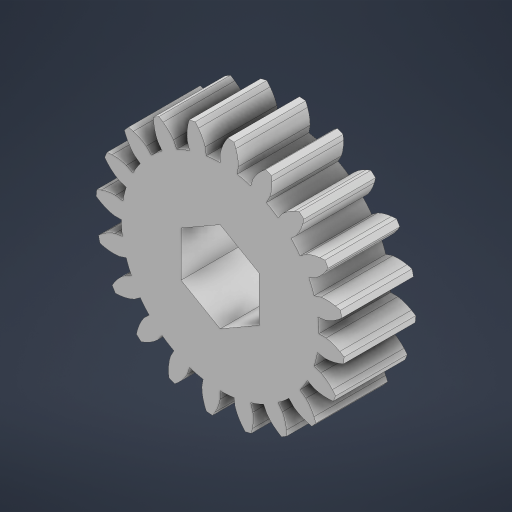
# Autodesk Inventor part: SpurGearTemplate
Saved by Autodesk Inventor 2024 (Build 280153000, 153)
## iProperties
Created: 2023-09-27
Part Number: SpurGearTemplate
Material: Generic
Document SubType Name: Modeling
Designer: avsar
Density: 1 g/cm^3
Appearance: Default
Author: avsar
Autodesk Inventor part; units mm, degrees
ref_plane "YZ Plane" through (0, 0, 0) normal (1, 0, 0) x (0, 1, 0)
ref_plane "XZ Plane" through (0, 0, 0) normal (0, 1, 0) x (-1, 0, 0)
ref_plane "XY Plane" through (0, 0, 0) normal (0, 0, 1) x (1, 0, 0)
sketch "Sketch1" plane through (0, 0, 0) normal (0, 0, 1) x (1, 0, 0)
  circle A0 centre (0, 0) radius 10 construction
  arc A1 (1.2256, 10.9315) -> (1.2111, 10.9331) centre (0, 0) ccw
  arc A2 (8.75, 0) -> (1.5067, 8.6193) centre (0, 0) ccw construction
  circle A3 centre (0, 0) radius 9 construction
  circle A4 centre (0, 0) radius 9.3969 construction
  line L0 (0, 0) -> (0, 9.3969) construction
  line L1 (0, 0) -> (4.6985, 8.138)
  line L2 (0, 0) -> (8.138, 4.6985)
  line L3 (0, 0) -> (9.3969, 0)
  line L4 (9.3969, 0) -> (9.3969, 14.7607) construction
  line L5 (8.138, 4.6985) -> (3.2178, 13.2205) construction
  line L6 (4.6985, 8.138) -> (0.4374, 10.5981) construction
  arc A5 (0.4374, 10.5981) -> (0, 9.3969) centre (3.6283, 8.7558) ccw
  arc A6 (3.2178, 13.2205) -> (0.9898, 11.41) centre (6.2054, 7.268) ccw construction
  arc A7 (9.3969, 14.7607) -> (3.2178, 13.2205) centre (9.7364, 0.2327) ccw construction
  line L7 (0, 0) -> (3.0902, 9.5106)
  line L8 (0, 0) -> (1.5643, 9.8769) construction
  arc A8 (1.5643, 9.8769) -> (0.1598, 9.9987) centre (0, 0) ccw construction
  line L9 (0.8642, 9.9626) -> (0, 0) construction
  arc A9 (3.0902, 9.5106) -> (0.1598, 9.9987) centre (0, 0) ccw construction
  arc A10 (1.6181, 9.2566) -> (1.394, 10.5151) centre (-2.0664, 9.2498) ccw
  arc A11 (1.394, 10.5151) -> (1.2256, 10.9315) centre (-4.8612, 8.2279) ccw
  arc A12 (-0.8932, 13.5771) -> (-6.7149, 16.1583) centre (-9.5509, 1.9057) ccw construction
  arc A13 (5.2789, 9.6506) -> (1.2256, 10.9315) centre (0, 0) ccw construction
  arc A14 (0.675, 10.9793) -> (5.2789, 9.6506) centre (0, 0) ccw construction
  arc A15 (0.9898, 11.41) -> (0.675, 10.9793) centre (6.2054, 7.268) ccw construction
  arc A16 (0.6896, 10.9784) -> (0.675, 10.9793) centre (0, 0) ccw
  arc A17 (1.2111, 10.9331) -> (0.6896, 10.9784) centre (0, 0) ccw
  arc A18 (1.2256, 10.9315) -> (-0.8932, 13.5771) centre (-4.8612, 8.2279) ccw construction
  arc A19 (0.675, 10.9793) -> (0.4374, 10.5981) centre (6.2054, 7.268) ccw
  line L10 (1.6181, 9.2566) -> (0, 0) construction
  arc A20 (0, 8.75) -> (8.75, 0) centre (0, 0) ccw construction
  arc A21 (1.5067, 8.6193) -> (0.7562, 8.7173) centre (0, 0) ccw
  arc A22 (0.7562, 8.7173) -> (0, 8.75) centre (0, 0) ccw
  line L11 (0, 9.3969) -> (0, 8.75)
  line L12 (1.5067, 8.6193) -> (1.6181, 9.2566)
  dimension "BaseCircle" = 18.7938
  dimension "PitchCircle" = 20
  dimension "AddendumCircle" = 22
  dimension "RootCircle" = 17.5
  dimension "ClearanceCircle" = 18
  dimension "InvoluteControl" = 90
  dimension "BaseCircleQuarterCircumference" = 14.7607
  dimension "d10" = 9.8404
  dimension "d11" = 4.9202
  dimension "CircularPitch" = 18
  constraints: 50 point on circle, 26 end point, 22 centre point, 7 symmetric about line, 5 coincident, 5 point on line, 2 collinear, 2 concentric, 2 tangent, 2 vertical, 1 line through centre, 1 vertical alignment, 18 other
  measures "PitchCircle" diameter of A0
  measures "AddendumCircle" diameter of A1
  measures "RootCircle" diameter of A2
  measures "ClearanceCircle" diameter of A3
  measures "BaseCircleQuarterCircumference" distance of L3.end L4.end
  measures "d10" distance of L2.end L5.end
  measures "d11" distance of L1.end L6.end
  measures "CircularPitch" angle of L7 L0
extrude "Extrusion1" add sketch "Sketch1" along normal mid plane 6.35
pattern_circular "Circular Pattern1" count 20 over 360 about axis through (0, 0, -10) along (0, 0, 1) of "Extrusion1"
sketch "Sketch2" plane through (0, 0, 0) normal (0, 0, 1) x (1, 0, 0)
  arc A0 (0, 8.75) -> (8.75, 0) centre (0, 0) ccw construction
  circle A1 centre (0, 0) radius 8.75
  arc A2 (8.75, 0) -> (1.5067, 8.6193) centre (0, 0) ccw construction
  constraints: 1 centre point, 1 coincident, 1 concentric
extrude "Extrusion2" add sketch "Sketch2" along normal mid plane 6.35
sketch "Sketch3" plane through (0, 0, 3.175) normal (0, 0, 1) x (1, 0, 0)
  circle A0 centre (0, 0) radius 4 construction
  line L0 (0, 0) -> (0, 4) construction
  line L1 (0, 4) -> (3.4641, 2)
  line L2 (3.4641, 2) -> (3.4641, -2)
  line L3 (3.4641, -2) -> (0, -4)
  line L4 (0, -4) -> (-3.4641, -2)
  line L5 (-3.4641, -2) -> (-3.4641, 2)
  line L6 (0, 4) -> (-3.4641, 2)
  dimension "d20" = 8
  constraints: 14 end point, 6 point on circle, 2 equal length, 2 parallel, 2 vertical, 1 centre point, 1 coincident
  measures "d20" diameter of A0
extrude "Extrusion3" cut sketch "Sketch3" against normal through all
equation "\"AddendumCircle\" = PitchCircle + 2 * Module"
equation "\"RootCircle\" = PitchCircle - 2.5 * Module"
equation "\"ClearanceCircle\" = PitchCircle - 2 * Module"
equation "\"BaseCircleQuarterCircumference\" = 0.785398 * BaseCircle"
equation "\"d10\" = 0.666667 * BaseCircleQuarterCircumference"
equation "\"d11\" = 0.333333 * BaseCircleQuarterCircumference"
equation "\"d18\" = GearThickness"
equation "\"PressureAngle\" = 20deg"
equation "\"Module\" = 1"
equation "\"GearThickness\" = 6.35"
body "Solid1"
